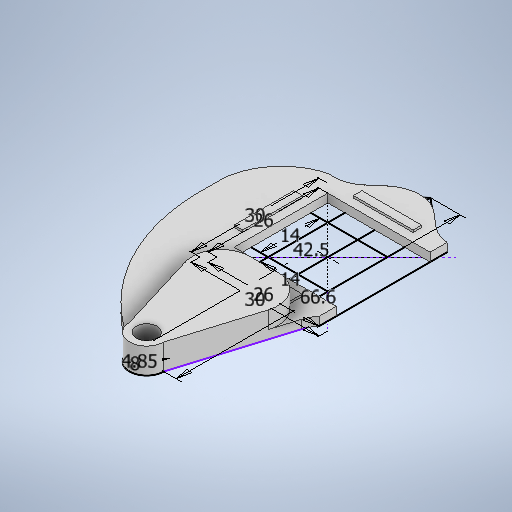
# Autodesk Inventor part: infeed plate
Saved by Autodesk Inventor 2025.1 (Build 291241000, 241)
## iProperties
Created: 2025-02-15
Part Number: infeed plate
Material: Generic
Document SubType Name: Modeling
Designer: m_kni
Density: 1 g/cm^3
Appearance: Default
Author: m_kni
## iProperties of the stored document infeed plate_3DPrint.ipt
Created: 2025-02-16
Part Number: infeed plate_3DPrint
Material: Generic
Document SubType Name: Modeling
Designer: m_kni
Density: 1 g/cm^3
Appearance: Default
Author: m_kni
Autodesk Inventor part; units mm, degrees
ref_plane "YZ Plane" through (0, 0, 0) normal (1, 0, 0) x (0, 1, 0)
ref_plane "XZ Plane" through (0, 0, 0) normal (0, 1, 0) x (-1, 0, 0)
ref_plane "XY Plane" through (0, 0, 0) normal (0, 0, 1) x (1, 0, 0)
sketch "Sketch1" plane through (0, 0, 0) normal (0, 1, 0) x (-1, 0, 0)
  circle A0 centre (0, 0) radius 2.425
  circle A1 centre (0, 0) radius 4
  line L0 (0, 0) -> (0, -66.6)
  line L1 (-13, -55.5) -> (13, -55.5)
  line L2 (13, -55.5) -> (13, -29.5)
  line L3 (13, -29.5) -> (-13, -29.5)
  line L4 (-13, -29.5) -> (-13, -55.5)
  line L5 (-13, -55.5) -> (13, -29.5) construction
  line L6 (13, -55.5) -> (-13, -29.5) construction
  line L7 (4, 0) -> (13, -29.5)
  line L8 (-4, 0) -> (-13, -29.5)
  line L9 (-13, -55.5) -> (0, -66.6)
  line L10 (13, -55.5) -> (0, -66.6)
  line L11 (-13, -57.5) -> (15, -57.5)
  line L12 (15, -57.5) -> (15, -27.5)
  line L13 (15, -27.5) -> (-13, -27.5)
  line L14 (-15, -57.5) -> (15, -27.5) construction
  line L15 (15, -57.5) -> (-15, -27.5) construction
  line L16 (-13, -29.5) -> (-13, -27.5)
  line L17 (-13, -55.5) -> (-13, -57.5)
  line L18 (-7, -49.5) -> (7, -49.5)
  line L19 (7, -49.5) -> (7, -35.5)
  line L20 (7, -35.5) -> (-7, -35.5)
  line L21 (-7, -35.5) -> (-7, -49.5)
  line L22 (-7, -49.5) -> (7, -35.5) construction
  line L23 (7, -49.5) -> (-7, -35.5) construction
  line L24 (9, -27.5) -> (9, -29.5)
  line L25 (-9, -27.5) -> (-9, -29.5)
  line L26 (13, -33.5) -> (15, -33.5)
  line L27 (13, -51.5) -> (15, -51.5)
  line L28 (9, -55.5) -> (9, -57.5)
  line L29 (-9, -55.5) -> (-9, -57.5)
  line L30 (7, -49.5) -> (7, -57.5)
  line L31 (-7, -49.5) -> (-7, -57.5)
  line L32 (7, -35.5) -> (7, -27.5)
  line L33 (-7, -35.5) -> (-7, -27.5)
  line L34 (7, -35.5) -> (15, -35.5)
  line L35 (7, -49.5) -> (15, -49.5)
  point P0 (0, -42.5)
  point P1 (-12.389831, -27.5)
  point P2 (12.389831, -27.5)
  point P3 (10.657658, -57.5)
  point P4 (-10.657658, -57.5)
  point P5 (7, -55.5)
  point P6 (-7, -55.5)
  point P7 (13, -49.5)
  point P8 (13, -35.5)
  point P9 (7, -29.5)
  point P10 (-7, -29.5)
  dimension "d0" = 4.85
  dimension "d1" = 8
  dimension "d2" = 66.6
  dimension "d3" = 42.5
  dimension "d4" = 26
  dimension "d5" = 26
  dimension "d6" = 30
  dimension "d7" = 30
  dimension "d8" = 14
  dimension "d9" = 14
  constraints: 72 end point, 22 point on line, 14 perpendicular, 6 midpoint, 5 parallel, 3 horizontal, 2 centre point, 2 coincident, 2 point on circle, 1 vertical
  measures "d0" diameter of A0
  measures "d1" diameter of A1
  measures "d2" distance of L0.start L0.end
  measures "d3" distance of point (0, -42.5) point (0, 0)
  measures "d4" distance of L3.end L2.end
  measures "d5" distance of L2.end L1.end
  measures "d6" distance of L15.end L12.end
  measures "d7" distance of L12.end L11.end
  measures "d8" distance of L20.end L19.end
  measures "d9" distance of L19.end L18.end
extrude "Extrusion1" add sketch "Sketch1" along normal blind 6 contours A1 | L7 L13 L0 A1 | A1 L0 L13 L8
extrude "Extrusion2" add sketch "Sketch1" along normal blind 2 contours L13 L12 L26 L2 L7 | L7 L3 L24 L13 | L13 L25 L3 L8 | L8 L16 L13 | L13 L32 L3 L0 | L0 L3 L33 L13 | L2 L34 L32 L3 | L24 L3 L32 L13 | L3 L33 L21 L31 L1 L4 | L13 L33 L3 L25 | L3 L32 L20 L0 | L0 L20 L33 L3 | L26 L12 L34 L2 | L1 L29 L11 L9 | L9 L11 L17 | L20 L19 L18 L0 | L0 L18 L21 L20 | L34 L12 L35 L2 | L2 L35 L19 L34 | L1 L31 L11 L29 | L11 L0 L9 | L18 L30 L1 L0 | L0 L1 L31 L18 | L35 L12 L27 L2 | L2 L1 L30 L35 | L1 L0 L11 L31 | L0 L11 L10 | L1 L30 L11 L0 | L27 L12 L11 L10 L2 | L11 L28 L1 L10 | L1 L28 L11 L30
extrude "Extrusion3" add sketch "Sketch1" along normal blind 2.5 contours L13 L32 L3 L0 | L0 L3 L33 L13 | L34 L12 L35 L2 | L1 L0 L11 L31 | L1 L30 L11 L0
sketch "Sketch2" plane through (0, 2, 0) normal (0, 1, 0) x (1, 0, 0)
  line L0 (13, 57.5) -> (10.657658, 57.5)
  line L1 (-15, 35.5) -> (-15, 27.5)
  line L2 (13, 57.5) -> (-15, 57.5)
  line L3 (-15, 57.5) -> (-15, 27.5)
  line L4 (-15, 27.5) -> (13, 27.5)
  line L5 (13, 27.5) -> (13, 57.5)
  line L6 (-13, 31.5) -> (13, 31.5)
  line L7 (13, 31.5) -> (13, 53.5)
  line L8 (13, 53.5) -> (-13, 53.5)
  line L9 (-13, 53.5) -> (-13, 31.5)
  line L10 (-13, 31.5) -> (13, 53.5) construction
  line L11 (13, 31.5) -> (-13, 53.5) construction
  line L12 (-11, 53.5) -> (-11, 31.5)
  point P0 (0, 0)
  point P1 (-15, 33.5)
  point P2 (0, 42.5)
  dimension "d16" = 22
  dimension "d17" = 2
  constraints: 22 end point, 4 parallel, 3 perpendicular, 3 point on line, 2 horizontal, 2 midpoint
  measures "d16" distance of L7.end L6.end
  measures "d17" distance of L12.start L8.end
extrude "Extrusion4" cut sketch "Sketch2" against normal blind 2.5 contours L5 L6 L12 L8
fillet "Fillet1" radius 6.7625 2 edges at (12.3898, 4, -27.5) (-12.3898, 4, -27.5)
sketch "Sketch3" plane through (0, 2, 0) normal (0, 1, 0) x (1, 0, 0)
  line L0 (-15, 40.5) -> (-26.283296, 40.5)
  line L1 (-26.283296, 40.5) -> (-26.283296, 44.5)
  line L2 (-26.283296, 44.5) -> (-15, 44.5)
  line L3 (26.283296, 40.5) -> (-26.283296, 44.5) construction
  line L4 (-26.283296, 40.5) -> (26.283296, 44.5) construction
  line L5 (-15, 57.5) -> (-15, 27.5)
  line L6 (-15, 40.5) -> (-15, 44.5)
  arc A0 (-4, 0) -> (4, 0) centre (0, 0) ccw
  arc A1 (-26.283296, 40.5) -> (-4, 0) centre (19.074711, 39.076006) ccw
  arc A2 (-15, 57.5) -> (-26.283296, 44.5) centre (-10.996696, 42.628704) ccw
  line L7 (7, 55.5) -> (-7, 55.5)
  line L8 (-13, 49.5) -> (-13, 35.5)
  line L9 (-11, 31.5) -> (-11, 53.5)
  line L10 (-11, 53.5) -> (-11, 31.5)
  line L11 (-11, 53.5) -> (-11, 31.5)
  line L12 (-11, 31.5) -> (-11, 53.5)
  line L13 (-15, 57.5) -> (-15, 49.5)
  line L14 (-15, 57.5) -> (-15, 27.5)
  line L15 (-15, 35.5) -> (-15, 27.5)
  line L16 (-15, 49.5) -> (-15, 35.5)
  line L17 (-11, 53.5) -> (13, 53.5)
  line L18 (13, 53.5) -> (13, 57.5)
  line L19 (13, 57.5) -> (10.657658, 57.5)
  line L20 (10.657658, 57.5) -> (0, 66.6)
  line L21 (0, 66.6) -> (-10.657658, 57.5)
  line L22 (-10.657658, 57.5) -> (-15, 57.5)
  line L23 (-15, 57.5) -> (-15, 49.5)
  line L24 (-13, 49.5) -> (-13, 35.5)
  line L25 (-15, 35.5) -> (-15, 27.5)
  line L26 (-15, 27.5) -> (-12.389831, 27.5)
  line L27 (-12.389831, 27.5) -> (-9.724658, 18.764158)
  arc A3 (-7, 26.369326) -> (-9.724658, 18.764158) centre (-3.25648, 20.7375) ccw
  line L28 (-7, 29.5) -> (7, 29.5)
  arc A4 (9.724658, 18.764158) -> (7, 26.369326) centre (3.25648, 20.7375) ccw
  line L29 (9.724658, 18.764158) -> (12.389831, 27.5)
  line L30 (12.389831, 27.5) -> (13, 27.5)
  line L31 (13, 27.5) -> (13, 31.5)
  line L32 (13, 31.5) -> (-11, 31.5)
  line L33 (-11, 31.5) -> (-11, 53.5)
  line L34 (-7, 57.5) -> (7, 57.5)
  line L35 (7, 55.5) -> (-7, 55.5)
  circle A5 centre (0, 0) radius 2.425
  line L36 (13, 53.5) -> (-11, 53.5)
  line L37 (-11, 53.5) -> (-11, 31.5)
  line L38 (-11, 31.5) -> (13, 31.5)
  line L39 (13, 27.5) -> (13, 31.5)
  line L40 (12.389831, 27.5) -> (13, 27.5)
  line L41 (4, 0) -> (12.389831, 27.5)
  arc A6 (-4, 0) -> (4, 0) centre (0, 0) ccw
  line L42 (-12.389831, 27.5) -> (-4, 0)
  line L43 (-15, 27.5) -> (-12.389831, 27.5)
  line L44 (-15, 57.5) -> (-15, 27.5)
  line L45 (-10.657658, 57.5) -> (-15, 57.5)
  line L46 (0, 66.6) -> (-10.657658, 57.5)
  line L47 (10.657658, 57.5) -> (0, 66.6)
  line L48 (13, 57.5) -> (10.657658, 57.5)
  line L49 (13, 53.5) -> (13, 57.5)
  line L50 (-9, 29.5) -> (9, 29.5)
  line L51 (-7, 29.5) -> (7, 29.5)
  line L52 (7, 29.5) -> (-7, 29.5)
  line L53 (13, 31.5) -> (-11, 31.5)
  line L54 (-11, 31.5) -> (13, 31.5)
  line L55 (-11, 31.5) -> (13, 31.5)
  line L56 (13, 31.5) -> (-11, 31.5)
  line L57 (12.389831, 27.5) -> (13, 27.5)
  line L58 (13, 27.5) -> (13, 31.5)
  line L59 (13, 27.5) -> (13, 31.5)
  line L60 (13, 27.5) -> (13, 31.5)
  line L61 (13, 27.5) -> (13, 31.5)
  line L62 (-13, 33.5) -> (-15, 33.5)
  line L63 (-15, 33.5) -> (-15, 27.5)
  line L64 (-9, 24.307288) -> (-9, 29.5)
  line L65 (-9, 29.5) -> (-9, 24.307288)
  line L66 (-9, 24.307288) -> (-9, 29.5)
  line L67 (-15, 27.5) -> (-12.389831, 27.5)
  line L68 (-15, 27.5) -> (-12.389831, 27.5)
  line L69 (-15, 27.5) -> (-12.389831, 27.5)
  line L70 (-12.389831, 27.5) -> (-9.724658, 18.764158)
  line L71 (-9, 55.5) -> (-9, 57.5)
  line L72 (-9, 57.5) -> (9, 57.5)
  line L73 (9, 57.5) -> (9, 55.5)
  line L74 (9, 29.5) -> (-9, 29.5)
  line L75 (7, 29.5) -> (-7, 29.5)
  arc A7 (-3.25648, 27.5) -> (-7, 26.369326) centre (-3.25648, 20.7375) ccw
  line L76 (3.25648, 27.5) -> (-3.25648, 27.5)
  arc A8 (7, 26.369326) -> (3.25648, 27.5) centre (3.25648, 20.7375) ccw
  line L77 (-15, 51.5) -> (-13, 51.5)
  line L78 (-15, 57.5) -> (-15, 51.5)
  line L79 (-10.657658, 57.5) -> (-15, 57.5)
  line L80 (-9, 29.5) -> (-9, 24.307288)
  line L81 (-11, 53.5) -> (13, 53.5)
  line L82 (13, 53.5) -> (13, 57.5)
  line L83 (0, 66.6) -> (-10.657658, 57.5)
  line L84 (10.657658, 57.5) -> (0, 66.6)
  line L85 (13, 57.5) -> (10.657658, 57.5)
  line L86 (-15, 27.5) -> (-12.389831, 27.5)
  line L87 (9, 29.5) -> (9, 24.307288)
  line L88 (9, 29.5) -> (9, 24.307288)
  line L89 (9, 29.5) -> (9, 24.307288)
  line L90 (9, 29.5) -> (9, 24.307288)
  line L91 (-10.657658, 57.5) -> (-15, 57.5)
  line L92 (-10.657658, 57.5) -> (-15, 57.5)
  line L93 (-10.657658, 57.5) -> (-15, 57.5)
  line L94 (13, 53.5) -> (13, 57.5)
  line L95 (13, 57.5) -> (10.657658, 57.5)
  line L96 (10.657658, 57.5) -> (0, 66.6)
  line L97 (0, 66.6) -> (-10.657658, 57.5)
  line L98 (-12.389831, 27.5) -> (-4, 0)
  circle A9 centre (0, 0) radius 2.425
  line L99 (3.25648, 27.5) -> (-3.25648, 27.5)
  circle A10 centre (0, 0) radius 2.425
  arc A11 (-9, 24.307288) -> (-9.724658, 18.764158) centre (-3.25648, 20.7375) ccw
  arc A12 (-3.25648, 27.5) -> (-9, 24.307288) centre (-3.25648, 20.7375) ccw
  arc A13 (9, 24.307288) -> (3.25648, 27.5) centre (3.25648, 20.7375) ccw
  arc A14 (9.724658, 18.764158) -> (9, 24.307288) centre (3.25648, 20.7375) ccw
  arc A15 (9.724658, 18.764158) -> (3.25648, 27.5) centre (3.25648, 20.7375) ccw
  arc A16 (9.724658, 18.764158) -> (3.25648, 27.5) centre (3.25648, 20.7375) ccw
  arc A17 (9.724658, 18.764158) -> (7, 26.369326) centre (3.25648, 20.7375) ccw
  arc A18 (7, 26.369326) -> (3.25648, 27.5) centre (3.25648, 20.7375) ccw
  line L100 (3.25648, 27.5) -> (-3.25648, 27.5)
  arc A19 (-3.25648, 27.5) -> (-9.724658, 18.764158) centre (-3.25648, 20.7375) ccw
  arc A20 (-3.25648, 27.5) -> (-9.724658, 18.764158) centre (-3.25648, 20.7375) ccw
  arc A21 (-3.25648, 27.5) -> (-7, 26.369326) centre (-3.25648, 20.7375) ccw
  arc A22 (-7, 26.369326) -> (-9.724658, 18.764158) centre (-3.25648, 20.7375) ccw
  line L101 (3.25648, 27.5) -> (-3.25648, 27.5)
  line L102 (3.25648, 27.5) -> (-3.25648, 27.5)
  line L103 (-12.389831, 27.5) -> (-9.724658, 18.764158)
  line L104 (-12.389831, 27.5) -> (-4, 0)
  line L105 (-9.724658, 18.764158) -> (-4, 0)
  line L106 (-9.724658, 18.764158) -> (-4, 0)
  line L107 (4, 0) -> (9.724658, 18.764158)
  arc A23 (-4, 0) -> (4, 0) centre (0, 0) ccw
  line L108 (13, 53.5) -> (-11, 53.5)
  line L109 (13, 53.5) -> (13, 57.5)
  line L110 (13, 53.5) -> (13, 57.5)
  line L111 (13, 53.5) -> (-11, 53.5)
  line L112 (-11, 53.5) -> (13, 53.5)
  line L113 (12.389831, 27.5) -> (13, 27.5)
  line L114 (9.724658, 18.764158) -> (12.389831, 27.5)
  line L115 (4, 0) -> (12.389831, 27.5)
  line L116 (12.389831, 27.5) -> (13, 27.5)
  line L117 (12.389831, 27.5) -> (13, 27.5)
  line L118 (-13, 35.5) -> (-13, 49.5)
  line L119 (-13, 49.5) -> (-13, 35.5)
  line L120 (-13, 35.5) -> (-13, 49.5)
  line L121 (-13, 33.5) -> (-15, 33.5)
  line L122 (-15, 33.5) -> (-13, 33.5)
  line L123 (-13, 51.5) -> (-15, 51.5)
  line L124 (-15, 33.5) -> (-13, 33.5)
  line L125 (-15, 51.5) -> (-13, 51.5)
  line L126 (-13, 51.5) -> (-15, 51.5)
  line L127 (-15, 49.5) -> (-15, 35.5)
  line L128 (-13, 35.5) -> (-13, 49.5)
  line L129 (-15, 51.5) -> (-15, 33.5)
  line L130 (-9, 57.5) -> (-9, 55.5)
  line L131 (9, 57.5) -> (-9, 57.5)
  line L132 (-7, 55.5) -> (7, 55.5)
  line L133 (7, 55.5) -> (-7, 55.5)
  line L134 (-7, 55.5) -> (7, 55.5)
  line L135 (9, 57.5) -> (9, 55.5)
  line L136 (9, 55.5) -> (9, 57.5)
  line L137 (-7, 55.5) -> (7, 55.5)
  line L138 (7, 57.5) -> (-7, 57.5)
  line L139 (-9, 55.5) -> (-9, 57.5)
  line L140 (-9, 57.5) -> (-9, 55.5)
  line L141 (-7, 57.5) -> (7, 57.5)
  line L142 (7, 57.5) -> (-7, 57.5)
  line L143 (0, 66.6) -> (-10.657658, 57.5)
  line L144 (0, 66.6) -> (-10.657658, 57.5)
  line L145 (9, 55.5) -> (9, 57.5)
  line L146 (13, 57.5) -> (10.657658, 57.5)
  line L147 (13, 57.5) -> (10.657658, 57.5)
  line L148 (10.657658, 57.5) -> (0, 66.6)
  line L149 (10.657658, 57.5) -> (0, 66.6)
  line L150 (4, 0) -> (9.724658, 18.764158)
  line L151 (4, 0) -> (12.389831, 27.5)
  line L152 (9.724658, 18.764158) -> (12.389831, 27.5)
  arc A24 (-3.25648, 27.5) -> (-9.724658, 18.764158) centre (-3.25648, 20.7375) ccw
  line L153 (-9.724658, 18.764158) -> (-4, 0)
  arc A25 (-4, 0) -> (4, 0) centre (0, 0) ccw
  line L154 (4, 0) -> (9.724658, 18.764158)
  arc A26 (9.724658, 18.764158) -> (3.25648, 27.5) centre (3.25648, 20.7375) ccw
  line L155 (3.25648, 27.5) -> (-3.25648, 27.5)
  circle A27 centre (0, 0) radius 2.425
  circle A28 centre (0, 0) radius 2.425
  circle A29 centre (0, 0) radius 2.425
  arc A30 (-4, 0) -> (4, 0) centre (0, 0) ccw
  arc A31 (-4, 0) -> (4, 0) centre (0, 0) ccw
  line L156 (-9, 55.5) -> (-9, 57.5)
  line L157 (13, 57.5) -> (-15, 57.5)
  line L158 (13, 55.5) -> (-13, 55.5)
  line L159 (9, 55.5) -> (9, 57.5)
  line L160 (13, 55.5) -> (13, 57.5)
  line L161 (7, 49.5) -> (-7, 49.5)
  line L162 (7, 35.5) -> (7, 49.5)
  line L163 (-7, 35.5) -> (7, 35.5)
  line L164 (7, 49.5) -> (-7, 35.5) construction
  line L165 (-7, 49.5) -> (7, 35.5) construction
  line L166 (13, 29.5) -> (13, 55.5)
  line L167 (-13, 29.5) -> (13, 29.5)
  line L168 (13, 55.5) -> (-13, 29.5) construction
  line L169 (-13, 55.5) -> (13, 29.5) construction
  line L170 (15, 57.5) -> (-15, 27.5) construction
  line L171 (-15, 57.5) -> (15, 27.5) construction
  line L172 (-15, 27.5) -> (13, 27.5)
  line L173 (9, 27.5) -> (9, 29.5)
  line L174 (-7, 49.5) -> (-7, 35.5)
  line L175 (-15, 57.5) -> (-15, 27.5)
  line L176 (-13, 55.5) -> (-13, 29.5)
  line L177 (-13, 51.5) -> (-15, 51.5)
  line L178 (13, 29.5) -> (13, 27.5)
  line L179 (13, 55.5) -> (0, 66.6)
  line L180 (-13, 55.5) -> (0, 66.6)
  circle A32 centre (0, 0) radius 2.425
  circle A33 centre (0, 0) radius 4
  line L181 (0, 0) -> (0, 66.6)
  line L182 (-4, 0) -> (-13, 29.5)
  line L183 (4, 0) -> (13, 29.5)
  line L184 (-9, 27.5) -> (-9, 29.5)
  line L185 (-13, 33.5) -> (-15, 33.5)
  line L186 (7, 55.5) -> (7, 57.5)
  line L187 (-7, 57.5) -> (-7, 55.5)
  line L188 (-15, 35.5) -> (-13, 35.5)
  line L189 (-13, 49.5) -> (-15, 49.5)
  line L190 (7, 29.5) -> (7, 26.369326)
  line L191 (-7, 29.5) -> (-7, 26.369326)
  line L192 (-15, 49.5) -> (-13, 49.5)
  line L193 (-13, 35.5) -> (-15, 35.5)
  line L194 (-7, 26.369326) -> (-7, 29.5)
  line L195 (7, 29.5) -> (7, 26.369326)
  line L196 (-7, 55.5) -> (-7, 57.5)
  line L197 (7, 57.5) -> (7, 55.5)
  point P0 (0, 42.5)
  dimension "d21" = 4
  constraints: 12 end point, 4 point on circle, 2 centre point, 2 midpoint, 2 point on line, 1 horizontal, 1 parallel, 1 perpendicular, 33 other
  measures "d21" distance of L0.end L1.end
extrude "Extrusion5" add sketch "Sketch3" against normal blind 2 contours L5 L26 L27 L42 A1 L0 | L0 L1 L2 L5 | L2 A2 L5
fillet "Fillet2" radius 8.35 4 edges at (-10.6577, 1, -57.5) (0, 1, -66.6) (10.6577, 1, -57.5) (12.3898, 1, -27.5)
fillet "Fillet3" radius 2 2 edges at (-9.6227, 2, -23.0183) (-6.8623, 2, -9.3821)
body "Solid1"
